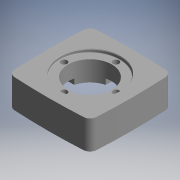
# Autodesk Inventor part: 1956846 EAMF-A-44C-60P(1A10)
Saved by Autodesk Inventor 2017.3 (Build 213256000, 256)
## iProperties
Part Number: 1956846 EAMF-A-44C-60P(1A10)
Material: Generic
Catalog Web Link: www.cadenas.de
Description: Adapter KGH.-Adapter KGH.
Vendor: FESTO
Document SubType Name: Modeling
Designer: partserver
Manufacturer: FESTO
Mass: 52.0199 g
Surface Area: 140.777 cm^2
Volume: 52.0199 cm^3
Density: 1 g/cm^3
Appearance: PSOLRGB-192-192-192
Category: PARTsolutions
Company: FESTO
Title: 1956846 EAMF-A-44C-60P(1A10)
Author: Cadenas PARTsolutions
Comments: Adapter KGH.
PSOL_IDENT_0: {$CADENAS_DATA\23d-libs\festo\parts\e\eamf\parts\eamf_a.prj},219 {VTYP=3D},{NB=1956846 EAMF-A-44C-60
PSOL_IDENT_1: P(1A10)},{LINA=1956846 EAMF-A-44C-60P(1A10)},{NN=Adapter KGH.},{DATE=10.06.2021 07:48:51},{GEOMDATE=
PSOL_IDENT_2: 10.06.2021 07:48:46},{VERSION=},{LINEID=970},{WBVAR=SVERS,S1},{WBNUMERIC=SVERS,S1}  {NB=1956846 EAMF
PSOL_IDENT_3: -A-44C-60P(1A10)},{LINA=1956846 EAMF-A-44C-60P(1A10)},{KT=DUMMY},{TNR=1956846},{TYP=EAMF-A-44C-60P},
PSOL_IDENT_4: {TNR1=1956326},{TNR2=-},{VERS=58},{TIF=0},{SVERS=1},{S1=0},{B1=0.000},{B2=0.000},{B3=0.000},{B4=0.00
PSOL_IDENT_5: 0},{B5=0.000},{D1=0.000},{D2=0.000},{D3=0.000},{D4=0.000},{D5=0.000},{D6=0.000},{D7=0.000},{D8=0.000
PSOL_IDENT_6: },{D9=0.000},{F1=0.000},{H1=0.000},{H2=0.000},{H3=0.000},{H4=0.000},{H5=0.000},{H6=0.000},{H7=0.000}
PSOL_IDENT_7: ,{L1=0.000},{L2=0.000},{L3=0.000},{L4=0.000},{L5=0.000},{L6=0.000},{R1=0.000},{R2=0.000},{T1=0.000},
PSOL_IDENT_8: {W=0.000},{W1=0.000},{W2=0.000},{SCH1=0.000}
NB: 1956846 EAMF-A-44C-60P(1A10)
NN: Adapter KGH.
NT: Adapter KGH.
NBSYN: $TNR. $TYP.($SVERS.A1$S1.)
LINA: 1956846 EAMF-A-44C-60P(1A10)
CATALOG: Festo
TNR: 1956846
TYP: EAMF-A-44C-60P
TNR1: 1956326
TNR2: -
VERS: 58
TIF: 0
SVERS: 1
S1: 0
B1: 0
B2: 0
B3: 0
B4: 0
B5: 0
D1: 0
D2: 0
D3: 0
D4: 0
D5: 0
D6: 0
D7: 0
D8: 0
D9: 0
F1: 0
H1: 0
H2: 0
H3: 0
H4: 0
H5: 0
H6: 0
H7: 0
L3: 0
L4: 0
L5: 0
L6: 0
R1: 0
R2: 0
T1: 0
W: 0
W1: 0
W2: 0
SCH1: 0
SUPPLIER: FESTO
ARTICLENO: 1956846 EAMF-A-44C-60P(1A10)
BOMINFO: 1956846 EAMF-A-44C-60P(1A10)
CREATOR: CADENAS GmbH
Autodesk Inventor part; units mm, degrees
sketch "Sketch_1" plane through (0, 0, 0) normal (0, 0, 1) x (1, 0, 0)
  arc A0 (-29.9895, 25.2782) -> (-29.9895, -25.2782) centre (419.3, 0) ccw
  arc A1 (-29.9895, -25.2782) -> (-25.2782, -29.9895) centre (-24.9973, -24.9973) ccw
  arc A2 (-25.2782, -29.9895) -> (25.2782, -29.9895) centre (0, 419.3) ccw
  arc A3 (25.2782, -29.9895) -> (29.9895, -25.2782) centre (24.9973, -24.9973) ccw
  arc A4 (29.9895, -25.2782) -> (29.9895, 25.2782) centre (-419.3, 0) ccw
  arc A5 (29.9895, 25.2782) -> (25.2782, 29.9895) centre (24.9973, 24.9973) ccw
  arc A6 (25.2782, 29.9895) -> (-25.2782, 29.9895) centre (0, -419.3) ccw
  arc A7 (-25.2782, 29.9895) -> (-29.9895, 25.2782) centre (-24.9973, 24.9973) ccw
  circle A8 centre (19, 0) radius 2.25
  circle A9 centre (0, 19) radius 2.25
  circle A10 centre (0, -19) radius 2.25
  circle A11 centre (-19, 0) radius 2.25
  constraints: 16 point on circle, 12 centre point
extrude "Extrusion1" add sketch "Sketch_1" against normal blind 21
sketch "Sketch_2" plane through (0, 0, 0) normal (1, 0, 0) x (0, 1, 0)
  line L0 (0, -21) -> (0, 0)
  line L1 (0, 0) -> (25.2887, 0)
  line L2 (25.2887, 0) -> (25, -0.5)
  line L3 (25, -0.5) -> (25, -3.7)
  arc A0 (24.7, -4) -> (25, -3.7) centre (24.7, -3.7) ccw
  line L4 (24.7, -4) -> (16, -4)
  line L5 (16, -4) -> (16, -18.7)
  line L6 (16, -18.7) -> (21.7, -18.7)
  arc A1 (22, -19) -> (21.7, -18.7) centre (21.7, -19) ccw
  line L7 (22, -19) -> (22, -20.5)
  line L8 (22, -20.5) -> (22.2887, -21)
  line L9 (22.2887, -21) -> (0, -21)
  line L10 (0, -21) -> (0, 0)
  constraints: 22 end point, 4 point on circle, 2 centre point
revolve "Revolution1" cut sketch "Sketch_2" angle 360 about axis through (0, 0, -21) along (0, 0, -1)
sketch "Sketch_3" plane through (0, 0, 0) normal (0, 0, 1) x (1, 0, 0)
  arc A0 (-19, 4) -> (-19, -4) centre (-19, 0) ccw
  line L0 (-19, -4) -> (-4, -4)
  line L1 (-4, -4) -> (-4, -19)
  arc A1 (-4, -19) -> (4, -19) centre (0, -19) ccw
  line L2 (4, -19) -> (4, -4)
  line L3 (4, -4) -> (19, -4)
  arc A2 (19, -4) -> (19, 4) centre (19, 0) ccw
  line L4 (19, 4) -> (4, 4)
  line L5 (4, 4) -> (4, 19)
  arc A3 (4, 19) -> (-4, 19) centre (0, 19) ccw
  line L6 (-4, 19) -> (-4, 4)
  line L7 (-4, 4) -> (-19, 4)
  constraints: 16 end point, 8 point on circle, 4 centre point
extrude "Extrusion2" cut sketch "Sketch_3" against normal blind 8
sketch "Sketch4" plane through (0, 0, 0) normal (0, 0, 1) x (1, 0, 0)
  point P0 (24.7487, 24.7487)
hole "Hole1" at (24.7487, 24.7487, 0) direction (0, 0, -1) diameter 3.242 depth 12.2188 tip angle 120 countersink diameter 4 countersink angle 90 thread size "M4x0.7" class "6H" standard "ISO Metric profile"
sketch "Sketch5" plane through (0, 0, 0) normal (0, 0, 1) x (1, 0, 0)
  point P0 (-24.7487, -24.7487)
hole "Hole2" at (-24.7487, -24.7487, 0) direction (0, 0, -1) diameter 3.242 depth 12.2188 tip angle 120 countersink diameter 4 countersink angle 90 thread size "M4x0.7" class "6H" standard "ISO Metric profile"
sketch "Sketch6" plane through (0, 0, 0) normal (0, 0, 1) x (1, 0, 0)
  point P0 (24.7487, -24.7487)
hole "Hole3" at (24.7487, -24.7487, 0) direction (0, 0, -1) diameter 3.242 depth 12.2188 tip angle 120 countersink diameter 4 countersink angle 90 thread size "M4x0.7" class "6H" standard "ISO Metric profile"
sketch "Sketch7" plane through (0, 0, 0) normal (0, 0, 1) x (1, 0, 0)
  point P0 (-24.7487, 24.7487)
hole "Hole4" at (-24.7487, 24.7487, 0) direction (0, 0, -1) diameter 3.242 depth 12.2188 tip angle 120 countersink diameter 4 countersink angle 90 thread size "M4x0.7" class "6H" standard "ISO Metric profile"
ref_plane "ANBAU_1_XY" through (0, 0, -21) normal (0, 0, 1) x (1, 0, 0)
ref_plane "ANBAU_1_YZ" through (0, 0, -21) normal (1, 0, 0) x (0, 1, 0)
ref_plane "ANBAU_1_ZX" through (0, 0, -21) normal (0, 1, 0) x (0, 0, 1)
ref_plane "ZYL_SCHRAUBE_1_1_XY" through (24.7487, 24.7487, 9) normal (0, 0, -1) x (1, 0, 0)
ref_plane "ZYL_SCHRAUBE_1_1_YZ" through (24.7487, 24.7487, 9) normal (1, 0, 0) x (0, -1, 0)
ref_plane "ZYL_SCHRAUBE_1_1_ZX" through (24.7487, 24.7487, 9) normal (0, -1, 0) x (0, 0, -1)
ref_plane "ZYL_SCHRAUBE_1_2_XY" through (-24.7487, 24.7487, 9) normal (0, 0, -1) x (1, 0, 0)
ref_plane "ZYL_SCHRAUBE_1_2_YZ" through (-24.7487, 24.7487, 9) normal (1, 0, 0) x (0, -1, 0)
ref_plane "ZYL_SCHRAUBE_1_2_ZX" through (-24.7487, 24.7487, 9) normal (0, -1, 0) x (0, 0, -1)
ref_plane "ZYL_SCHRAUBE_1_3_XY" through (-24.7487, -24.7487, 9) normal (0, 0, -1) x (1, 0, 0)
ref_plane "ZYL_SCHRAUBE_1_3_YZ" through (-24.7487, -24.7487, 9) normal (1, 0, 0) x (0, -1, 0)
ref_plane "ZYL_SCHRAUBE_1_3_ZX" through (-24.7487, -24.7487, 9) normal (0, -1, 0) x (0, 0, -1)
ref_plane "ZYL_SCHRAUBE_1_4_XY" through (24.7487, -24.7487, 9) normal (0, 0, -1) x (1, 0, 0)
ref_plane "ZYL_SCHRAUBE_1_4_YZ" through (24.7487, -24.7487, 9) normal (1, 0, 0) x (0, -1, 0)
ref_plane "ZYL_SCHRAUBE_1_4_ZX" through (24.7487, -24.7487, 9) normal (0, -1, 0) x (0, 0, -1)
ref_plane "ZYL_SCHRAUBE_2_1_XY" through (19, 0, -8) normal (0, 0, -1) x (1, 0, 0)
ref_plane "ZYL_SCHRAUBE_2_1_YZ" through (19, 0, -8) normal (1, 0, 0) x (0, -1, 0)
ref_plane "ZYL_SCHRAUBE_2_1_ZX" through (19, 0, -8) normal (0, -1, 0) x (0, 0, -1)
ref_plane "ZYL_SCHRAUBE_2_2_XY" through (0, 19, -8) normal (0, 0, -1) x (1, 0, 0)
ref_plane "ZYL_SCHRAUBE_2_2_YZ" through (0, 19, -8) normal (1, 0, 0) x (0, -1, 0)
ref_plane "ZYL_SCHRAUBE_2_2_ZX" through (0, 19, -8) normal (0, -1, 0) x (0, 0, -1)
ref_plane "ZYL_SCHRAUBE_2_3_XY" through (-19, 0, -8) normal (0, 0, -1) x (1, 0, 0)
ref_plane "ZYL_SCHRAUBE_2_3_YZ" through (-19, 0, -8) normal (1, 0, 0) x (0, -1, 0)
ref_plane "ZYL_SCHRAUBE_2_3_ZX" through (-19, 0, -8) normal (0, -1, 0) x (0, 0, -1)
ref_plane "ZYL_SCHRAUBE_2_4_XY" through (0, -19, -8) normal (0, 0, -1) x (1, 0, 0)
ref_plane "ZYL_SCHRAUBE_2_4_YZ" through (0, -19, -8) normal (1, 0, 0) x (0, -1, 0)
ref_plane "ZYL_SCHRAUBE_2_4_ZX" through (0, -19, -8) normal (0, -1, 0) x (0, 0, -1)
body "Solid1"
